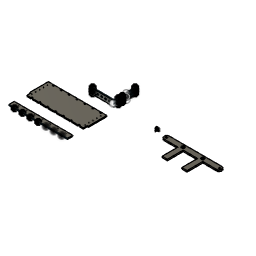
Supporto Netgear v27 (Autodesk Fusion 360 design; units mm, degrees)
Autodesk Fusion 360 part; units mm, degrees
sketch "Schizzo1" plane through (0, 0, 0) normal (0, 0, 1) x (1, 0, 0)
  line L0 (10, 5.25) -> (18, 5.25)
  line L1 (18, 5.25) -> (18, -2.75)
  line L2 (18, -2.75) -> (10, -2.75)
  line L3 (10, -2.75) -> (10, 5.25)
  line L4 (14, 5.25) -> (14, -2.75) construction
  line L5 (10, 1.25) -> (18, 1.25) construction
  circle A0 centre (14, 1.25) radius 2
  line L6 (10, 3.25) -> (18, 3.25) construction
  line L7 (12, 5.25) -> (12, -2.75) construction
  line L8 (12, 5.25) -> (10, 3.25)
  line L9 (16, 5.25) -> (18, 3.25)
  line L10 (16, -2.75) -> (18, -0.75)
  line L11 (12, -2.75) -> (10, -0.75)
  line L12 (21, -0.5) -> (7, -0.5)
  line L13 (7, -0.5) -> (7, 3)
  line L14 (7, 3) -> (21, 3)
  line L15 (21, 3) -> (21, -0.5)
  line L16 (21, -0.5) -> (7, 3) construction
  line L17 (7, -0.5) -> (21, 3) construction
  line L18 (61.544, 0) -> (261.544, 0)
  line L19 (261.544, 0) -> (261.544, -20)
  line L20 (261.544, -20) -> (61.544, -20)
  line L21 (61.544, -20) -> (61.544, 0)
  line L22 (61.544, -10) -> (261.544, -10) construction
  line L23 (124.044, 0) -> (124.044, -20) construction
  line L24 (199.044, 0) -> (199.044, -20) construction
  line L25 (124.044, -10) -> (161.544, -10) construction
  line L26 (161.544, -10) -> (199.044, -10) construction
  circle A1 centre (124.044, -10) radius 3.1
  line L27 (120.944, -10) -> (120.944, -6.9)
  arc A2 (127.144, -6.9) -> (120.944, -6.9) centre (124.044, -6.9) ccw
  line L28 (127.144, -6.9) -> (127.144, -10)
  line L29 (161.544, 0) -> (161.544, -20) construction
  line L30 (124.044, -10) -> (120.944, -10) construction
  line L31 (124.044, -10) -> (127.144, -10) construction
  line L32 (120.944, -10) -> (120.944, -13.1)
  arc A3 (120.944, -13.1) -> (127.144, -13.1) centre (124.044, -13.1) ccw
  line L33 (127.144, -13.1) -> (127.144, -10)
  line L34 (195.944, -13.1) -> (195.944, -10)
  arc A4 (195.944, -13.1) -> (202.144, -13.1) centre (199.044, -13.1) ccw
  line L35 (202.144, -10) -> (202.144, -13.1)
  arc A5 (202.144, -6.9) -> (195.944, -6.9) centre (199.044, -6.9) ccw
  line L36 (202.144, -10) -> (202.144, -6.9)
  line L37 (195.944, -6.9) -> (195.944, -10)
  circle A6 centre (124.044, -10) radius 6.2
  circle A7 centre (199.044, -10) radius 6.2
  circle A8 centre (59.944, -10) radius 3.4
  circle A9 centre (263.144, -10) radius 3.4
  arc A10 (61.544, 0) -> (61.544, -20) centre (61.544, -10) ccw
  arc A11 (261.544, -20) -> (261.544, 0) centre (261.544, -10) ccw
  line L38 (114.044, -20) -> (134.044, -20)
  line L39 (134.044, -20) -> (134.044, -80)
  line L40 (134.044, -80) -> (114.044, -80)
  line L41 (114.044, -80) -> (114.044, -20)
  line L42 (189.044, -20) -> (189.044, -80)
  line L43 (209.044, -80) -> (209.044, -20)
  line L44 (189.044, -80) -> (209.044, -80)
  line L45 (209.044, -20) -> (189.044, -20)
  line L46 (63.994, -5.95) -> (55.894, -5.95)
  line L47 (55.894, -5.95) -> (55.894, -14.05)
  line L48 (55.894, -14.05) -> (63.994, -14.05)
  line L49 (63.994, -14.05) -> (63.994, -5.95)
  line L50 (63.994, -5.95) -> (55.894, -14.05) construction
  line L51 (55.894, -5.95) -> (63.994, -14.05) construction
  line L52 (267.194, -5.95) -> (267.194, -14.05)
  line L53 (267.194, -14.05) -> (259.094, -14.05)
  line L54 (259.094, -14.05) -> (259.094, -5.95)
  line L55 (259.094, -5.95) -> (267.194, -5.95)
  line L56 (-150, 0) -> (-146, 0)
  line L57 (-146, 0) -> (-146, 86)
  line L58 (-146, 86) -> (-150, 86)
  line L59 (-150, 86) -> (-150, 0)
  line L60 (-146, 0) -> (-236, 0)
  line L61 (-236, 0) -> (-236, -4)
  line L62 (-236, -4) -> (-146, -4)
  line L63 (-146, -4) -> (-146, 0)
  line L64 (-150, 15) -> (-165, 0)
  line L65 (-350.1087, -50) -> (-330.1087, -50) construction
  line L66 (-330.1087, -50) -> (-330.1087, -136) construction
  line L67 (-330.1087, -136) -> (-350.1087, -136) construction
  line L68 (-350.1087, -136) -> (-350.1087, -50) construction
  line L69 (-340.1087, -50) -> (-340.1087, -136) construction
  line L70 (-350.1087, -93) -> (-330.1087, -93) construction
  line L71 (-350.1087, -50) -> (-126.9087, -50)
  line L72 (-126.9087, -50) -> (-126.9087, -136)
  line L73 (-126.9087, -136) -> (-350.1087, -136)
  line L74 (-350.1087, -136) -> (-350.1087, -50)
  line L75 (-146.9087, -50) -> (-126.9087, -50) construction
  line L76 (-126.9087, -50) -> (-126.9087, -136) construction
  line L77 (-126.9087, -136) -> (-146.9087, -136) construction
  line L78 (-146.9087, -136) -> (-146.9087, -50) construction
  line L79 (-136.9087, -50) -> (-136.9087, -136) construction
  line L80 (-146.9087, -93) -> (-126.9087, -93) construction
  circle A12 centre (-340.1087, -93) radius 1.4
  line L81 (-330.1087, -78) -> (-350.1087, -78) construction
  line L82 (-330.1087, -63) -> (-350.1087, -63) construction
  circle A13 centre (-340.1087, -78) radius 1.4
  circle A14 centre (-340.1087, -63) radius 1.4
  circle A15 centre (-340.1087, -123) radius 1.4
  circle A16 centre (-340.1087, -108) radius 1.4
  line L83 (-238.5087, -50) -> (-238.5087, -136) construction
  line L84 (-330.1087, -93) -> (-146.9087, -93) construction
  circle A17 centre (-136.9087, -63) radius 1.4
  circle A18 centre (-136.9087, -78) radius 1.4
  circle A19 centre (-136.9087, -93) radius 1.4
  circle A20 centre (-136.9087, -108) radius 1.4
  circle A21 centre (-136.9087, -123) radius 1.4
  line L85 (-350.1087, -134) -> (-126.9087, -134) construction
  line L86 (-268.5087, -136) -> (-268.5087, -50) construction
  line L87 (-298.5087, -136) -> (-298.5087, -50) construction
  line L88 (-328.5087, -50) -> (-328.5087, -136) construction
  circle A22 centre (-328.5087, -134) radius 1.4
  circle A23 centre (-298.5087, -134) radius 1.4
  circle A24 centre (-268.5087, -134) radius 1.4
  circle A25 centre (-238.5087, -134) radius 1.4
  circle A26 centre (-328.5087, -134) radius 3
  circle A27 centre (-298.5087, -134) radius 3
  circle A28 centre (-268.5087, -134) radius 3
  circle A29 centre (-238.5087, -134) radius 3
  circle A30 centre (-148.5087, -134) radius 3
  circle A31 centre (-148.5087, -134) radius 1.4
  circle A32 centre (-178.5087, -134) radius 1.4
  circle A33 centre (-178.5087, -134) radius 3
  circle A34 centre (-208.5087, -134) radius 3
  circle A35 centre (-208.5087, -134) radius 1.4
  circle A36 centre (-328.5087, -52) radius 3
  circle A37 centre (-328.5087, -52) radius 1.4
  circle A38 centre (-298.5087, -52) radius 3
  circle A39 centre (-298.5087, -52) radius 1.4
  circle A40 centre (-268.5087, -52) radius 3
  circle A41 centre (-268.5087, -52) radius 1.4
  circle A42 centre (-238.5087, -52) radius 3
  circle A43 centre (-238.5087, -52) radius 1.4
  circle A44 centre (-208.5087, -52) radius 3
  circle A45 centre (-208.5087, -52) radius 1.4
  circle A46 centre (-178.5087, -52) radius 1.4
  circle A47 centre (-178.5087, -52) radius 3
  circle A48 centre (-148.5087, -52) radius 1.4
  circle A49 centre (-148.5087, -52) radius 3
  line L89 (-350.1087, -121) -> (-126.9087, -121) construction
  line L90 (-350.1087, -121) -> (-346.1087, -121)
  line L91 (-346.1087, -121) -> (-346.1087, -136)
  line L92 (-346.1087, -136) -> (-350.1087, -136)
  line L93 (-350.1087, -136) -> (-350.1087, -121)
  line L94 (-130.9087, -121) -> (-130.9087, -136)
  line L95 (-126.9087, -121) -> (-130.9087, -121)
  line L96 (-350.1087, -180) -> (-126.9087, -180)
  line L97 (-126.9087, -180) -> (-126.9087, -200)
  line L98 (-126.9087, -200) -> (-350.1087, -200)
  line L99 (-350.1087, -200) -> (-350.1087, -180)
  line L100 (-126.9087, -136) -> (-126.9087, -180) construction
  line L101 (-350.1087, -136) -> (-350.1087, -180) construction
  line L102 (15.75, -5.75) -> (12.25, -5.75)
  line L103 (12.25, -5.75) -> (12.25, 8.25)
  line L104 (12.25, 8.25) -> (15.75, 8.25)
  line L105 (15.75, 8.25) -> (15.75, -5.75)
  line L106 (15.75, -5.75) -> (12.25, 8.25) construction
  line L107 (12.25, -5.75) -> (15.75, 8.25) construction
  arc A50 (15.75, 8.25) -> (12.25, 8.25) centre (14, 8.25) ccw
  arc A51 (12.25, -5.75) -> (15.75, -5.75) centre (14, -5.75) ccw
  arc A52 (21, -0.5) -> (21, 3) centre (21, 1.25) ccw
  arc A53 (7, 3) -> (7, -0.5) centre (7, 1.25) ccw
  line L108 (124.044, -20) -> (124.044, -80) construction
  point P0 (14, 1.25)
  point P1 (59.944, -10)
  point P2 (14, 1.25)
  point P3 (124.044, -3.8)
  point P4 (124.044, -16.2)
  dimension "d1" = 8
  dimension "d2" = 8
  dimension "d3" = 4
  dimension "d8" = 2
  dimension "d9" = 2
  dimension "d10" = 14
  dimension "d11" = 3.5
  dimension "d12" = 200
  dimension "d13" = 20
  dimension "d14" = 75
  dimension "d15" = 6.2
  dimension "d28" = 6.8
  dimension "d29" = 101.6
  dimension "d30" = 203.2
  dimension "d31" = 20
  dimension "d32" = 60
  dimension "d63" = 8.1
  dimension "d64" = 8.1
  dimension "d67" = 4
  dimension "d69" = 90
  dimension "d70" = 4
  dimension "d117" = 20
  dimension "d118" = 86
  dimension "d119" = 20
  dimension "d121" = 86
  dimension "d122" = 203.2
  dimension "d125" = 90
  dimension "d126" = 2.8
  dimension "d127" = 15
  dimension "d128" = 15
  dimension "d129" = 2.8
  dimension "d130" = 2.8
  dimension "d131" = 2
  dimension "d132" = 30
  dimension "d133" = 30
  dimension "d134" = 30
  dimension "d135" = 2.8
  dimension "d136" = 2.8
  dimension "d137" = 2.8
  dimension "d138" = 2.8
  dimension "d139" = 6
  dimension "d140" = 6
  dimension "d141" = 6
  dimension "d142" = 6
  dimension "d148" = 15
  dimension "d149" = 15
  dimension "d150" = 15
  dimension "d151" = 4
  dimension "d162" = 20
  dimension "d172" = 3.5
  dimension "d173" = 14
  dimension "d180" = 12.4
  constraint horizontal L0
  constraint vertical L1
  constraint horizontal L2
  constraint vertical L3
  constraint midpoint L0 L4.start
  constraint midpoint L2 L4.end
  constraint midpoint L3 L5.start
  constraint midpoint L1 L5.end
  constraint midpoint L4 P2
  constraint coincident L3 L6.start
  constraint coincident L1 L6.end
  constraint perpendicular L1 L6
  constraint coincident L0 L7.start
  constraint coincident L2 L7.end
  constraint perpendicular L2 L7
  constraint symmetric L4 L6.start L6.end
  constraint symmetric L4 L7.start L9.start
  constraint symmetric L5 L6.start L11.end
  constraint symmetric L5 L7.start L7.end
  constraint symmetric L5 L9.start L10.start
  constraint symmetric L5 L6.end L10.end
  constraint horizontal L12
  constraint perpendicular L12 L13
  constraint parallel L12 L14
  constraint parallel L13 L15
  constraint coincident L16 P2
  constraint coincident L17 P2
  constraint coincident P2 P0
  constraint horizontal L18
  constraint vertical L19
  constraint horizontal L20
  constraint vertical L21
  constraint midpoint L21 L22.start
  constraint midpoint L19 L22.end
  constraint coincident L18 L23.start
  constraint coincident L20 L23.end
  constraint perpendicular L20 L23
  constraint coincident L18 L24.start
  constraint coincident L20 L24.end
  constraint perpendicular L20 L24
  constraint coincident L23 L25.start
  constraint coincident L24 L26.end
  constraint perpendicular L24 L26
  constraint equal L25 L26
  constraint midpoint L23 L25.start
  constraint parallel L23 L27
  constraint tangent L27 A2
  constraint tangent A2 L28
  constraint parallel L23 L28
  constraint coincident L22 L27.start
  constraint coincident A1 L27.start
  constraint tangent A1 L28
  constraint coincident A1 A2.centre
  constraint collinear L22 L25
  constraint midpoint L18 L29.start
  constraint perpendicular L22 L29
  constraint coincident L25.end L29
  constraint coincident L25.start A1.centre
  constraint coincident A1 L28.end
  constraint coincident L22 L28.end
  constraint coincident L28.end L31.end
  constraint symmetric L22 L27.start L30.end
  constraint symmetric L22 L27.end L32.end
  constraint symmetric L22 A2.start A3.end
  constraint symmetric L22 A2 A3
  constraint symmetric L22 L28.end L31.end
  constraint symmetric L27.start L29 L35.start
  constraint symmetric L27.end L29 A5.start
  constraint symmetric A2.start L29 A5.end
  constraint symmetric A2 L29 A5
  constraint symmetric L28.end L29 L34.end
  constraint symmetric L29 L27.start L35.start
  constraint symmetric L29 L32.end A4.end
  constraint symmetric L29 A3.end L34.start
  constraint symmetric L29 A3 A4
  constraint symmetric L29 L28.end L34.end
  constraint tangent A2 A6
  constraint symmetric L29 A6 A7
  constraint coincident L22 P1
  constraint symmetric L29 A8 A9
  constraint tangent L18 A10
  constraint symmetric L18.start L29 L18.end
  constraint symmetric L20.end L29 L19.end
  constraint symmetric L29 A10 A11
  constraint coincident L20 L29.end
  constraint horizontal L38
  constraint vertical L39
  constraint horizontal L40
  constraint vertical L41
  constraint collinear L20 L38
  constraint symmetric L29 L38.start L43.end
  constraint symmetric L29 L38.end L42.start
  constraint symmetric L29 L39.end L42.end
  constraint symmetric L29 L40.end L43.start
  constraint horizontal L46
  constraint perpendicular L46 L47
  constraint parallel L46 L48
  constraint parallel L47 L49
  constraint coincident L50 P1
  constraint coincident L51 P1
  constraint coincident P1 A8.centre
  constraint symmetric L29 L46.start L54.end
  constraint symmetric L29 L46.end L52.start
  constraint symmetric L29 L47.end L52.end
  constraint symmetric L29 L48.end L53.end
  constraint horizontal L56
  constraint vertical L57
  constraint horizontal L58
  constraint vertical L59
  constraint horizontal L60
  constraint vertical L61
  constraint horizontal L62
  constraint vertical L63
  constraint coincident L59 L64.start
  constraint coincident L60 L64.end
  constraint horizontal L65
  constraint vertical L66
  constraint horizontal L67
  constraint vertical L68
  constraint midpoint L65 L69.start
  constraint midpoint L67 L69.end
  constraint midpoint L68 L70.start
  constraint midpoint L66 L70.end
  constraint horizontal L71
  constraint vertical L72
  constraint horizontal L73
  constraint vertical L74
  constraint collinear L67 L73
  constraint horizontal L75
  constraint vertical L76
  constraint horizontal L77
  constraint vertical L78
  constraint midpoint L75 L79.start
  constraint midpoint L77 L79.end
  constraint midpoint L78 L80.start
  constraint midpoint L76 L80.end
  constraint collinear L72 L76
  constraint midpoint L70 A12.centre
  constraint coincident L66 L81.start
  constraint coincident L74 L81.end
  constraint perpendicular L74 L81
  constraint coincident L66 L82.start
  constraint coincident L68 L82.end
  constraint perpendicular L68 L82
  constraint midpoint L81 A13.centre
  constraint midpoint L82 A14.centre
  constraint symmetric L70 A13 A16
  constraint symmetric L70 A14 A15
  constraint midpoint L71 L83.start
  constraint midpoint L73 L83.end
  constraint perpendicular L78 L84
  constraint symmetric A12 L83 A19
  constraint symmetric A13 L83 A18
  constraint symmetric A14 L83 A17
  constraint symmetric A15 L83 A21
  constraint symmetric A16 L83 A20
  constraint coincident L74 L85.start
  constraint coincident L76 L85.end
  constraint perpendicular L76 L85
  constraint coincident L73 L86.start
  constraint coincident L71 L86.end
  constraint perpendicular L71 L86
  constraint coincident L73 L87.start
  constraint coincident L71 L87.end
  constraint perpendicular L71 L87
  constraint coincident L71 L88.start
  constraint coincident L73 L88.end
  constraint perpendicular L73 L88
  constraint coincident L88 A22.centre
  constraint coincident L85 A22.centre
  constraint coincident L87 A23.centre
  constraint coincident L85 A23.centre
  constraint coincident L85 A24.centre
  constraint coincident L86 A24.centre
  constraint midpoint L85 A25.centre
  constraint concentric A22 A26
  constraint concentric A23 A27
  constraint concentric A24 A28
  constraint concentric A25 A29
  constraint symmetric L83 A22 A31
  constraint symmetric L83 A23 A32
  constraint symmetric L83 A24 A35
  constraint symmetric L83 A26 A30
  constraint symmetric L83 A27 A33
  constraint symmetric L83 A28 A34
  constraint symmetric L84 A22 A37
  constraint symmetric L84 A23 A39
  constraint symmetric L84 A24 A41
  constraint symmetric L84 A25 A43
  constraint symmetric L84 A26 A36
  constraint symmetric L84 A27 A38
  constraint symmetric L84 A28 A40
  constraint symmetric L84 A29 A42
  constraint symmetric L84 A30 A49
  constraint symmetric L84 A31 A48
  constraint symmetric L84 A32 A46
  constraint symmetric L84 A33 A47
  constraint symmetric L84 A34 A44
  constraint symmetric L84 A35 A45
  constraint coincident L74 L89.start
  constraint coincident L76 L89.end
  constraint perpendicular L76 L89
  constraint horizontal L90
  constraint vertical L91
  constraint horizontal L92
  constraint vertical L93
  constraint symmetric L83 L89.start L89.end
  constraint symmetric L83 L90.end L94.start
  constraint symmetric L83 L91.end L94.end
  constraint horizontal L96
  constraint vertical L97
  constraint horizontal L98
  constraint vertical L99
  constraint perpendicular L77 L100
  constraint coincident L96.end L97.start
  constraint perpendicular L92 L101
  constraint coincident L96.start L99.end
  constraint horizontal L102
  constraint perpendicular L102 L103
  constraint parallel L102 L104
  constraint parallel L103 L105
  constraint coincident L106 P2
  constraint coincident L107 P2
  constraint tangent L105 A50
  constraint tangent L105 A51
  constraint tangent L14 A52
  constraint tangent L12 A53
  constraint midpoint L38 L23.end
  constraint midpoint L40 L108.end
  constraint collinear L23 L108
  constraint midpoint A2 P3
  constraint midpoint A3 P4
  measures "d1" distance of L0.start L0.end
  measures "d2" distance of L0.start L2.end
  measures "d3" diameter of A0
  measures "d8" distance of L0 L6
  measures "d9" distance of L3 L7
  measures "d10" distance of L13.end L14.end
  measures "d11" distance of L12.end L13.end
  measures "d12" distance of L18.start L18.end
  measures "d13" distance of L18.start L20.end
  measures "d14" distance of L23 L24
  measures "d15" diameter of A1
  measures "d28" diameter of A8
  measures "d29" distance of L29 P1
  measures "d30" distance of P1 A9.centre
  measures "d31" distance of L38.start L38.end
  measures "d32" distance of L38.start L40.end
  measures "d63" distance of L47.end L48.end
  measures "d64" distance of L46.end L47.end
  measures "d67" distance of L56.start L56.end
  measures "d69" distance of L56.end L60.end
  measures "d70" distance of L56.end L62.end
  measures "d117" distance of L65.start L65.end
  measures "d118" distance of L65.start L67.end
  measures "d119" distance of L75.start L71.end
  measures "d121" distance of L71.end L72.end
  measures "d122" distance of L69 L79
  measures "d125" distance of L57.end L62.end
  measures "d126" diameter of A12
  measures "d127" distance of L81 L82
  measures "d128" distance of L70 L81
  measures "d129" diameter of A13
  measures "d130" diameter of A14
  measures "d131" distance of L73 L85
  measures "d132" distance of L83 L86
  measures "d133" distance of L86 L87
  measures "d134" distance of L87 L88
  measures "d135" diameter of A22
  measures "d136" diameter of A23
  measures "d137" diameter of A24
  measures "d138" diameter of A25
  measures "d139" diameter of A26
  measures "d140" diameter of A27
  measures "d141" diameter of A28
  measures "d142" diameter of A29
  measures "d148" distance of L56.start L64.end
  measures "d149" distance of L56.start L64.start
  measures "d150" distance of L67 L89
  measures "d151" distance of L89.start L90.end
  measures "d162" distance of L96.start L98.end
  measures "d172" distance of L103.end L104.end
  measures "d173" distance of L102.end L103.end
  measures "d180" distance of P3 P4
extrude "Estrusione1" add sketch "Schizzo1" along normal blind 2.8 contours L0 L3 L8 L14 L103 | L0 L103 L104 L105 | L0 A0 L14 L103 L105 | L3 A0 L12 L14 L103 | L3 L12 L13 L14 | L0 L1 L9 L14 L105 | A0 L14 L103 | L104 A50 | L2 L3 L11 L12 L103 | L13 A53 | A0 L14 L105 | L1 A0 L12 L14 L105 | A0 L12 L103 | L2 A0 L12 L103 L105 | L1 L12 L14 L15 | L2 L102 L103 L105 | L1 L2 L10 L12 L105 | L15 A52 | A0 L12 L105 | L102 A51 makes body 1
extrude "Estrusione2" add sketch "Schizzo1" along normal blind 6 contours A0 L12 L14 L103 L105 | A0 L14 | A0 L103 | A0 L105 | A0 L12 bodies 1
sketch "Schizzo2" plane through (0, 0, 6) normal (0, 0, 1) x (-1, 0, 0)
  line L0 (-17.5, -0.65) -> (-10.5, -0.65)
  line L1 (-10.5, -0.65) -> (-10.5, -1.85)
  line L2 (-10.5, -1.85) -> (-17.5, -1.85)
  line L3 (-17.5, -1.85) -> (-17.5, -0.65)
  line L4 (-17.5, -0.65) -> (-10.5, -1.85) construction
  line L5 (-10.5, -0.65) -> (-17.5, -1.85) construction
  circle A0 centre (-14, -1.25) radius 3 construction
  circle A1 centre (-14, -1.25) radius 2 construction
  line L6 (-11, -1.25) -> (-11, 1.75) construction
  line L7 (-17, -1.25) -> (-17, 1.75) construction
  line L8 (-11, 1.75) -> (-17, 1.75)
  line L9 (-11, -1.25) -> (-17, -1.25) construction
  line L10 (-14, 1.75) -> (-14.0003, -4.25) construction
  line L11 (-11, -4.25) -> (-17, -4.25)
  arc A2 (-17, 1.75) -> (-17, -4.25) centre (-17, -1.25) ccw
  arc A3 (-11, -4.25) -> (-11, 1.75) centre (-11, -1.25) ccw
  point P0 (-14, -1.25)
  dimension "d24" = 7
  dimension "d25" = 1.2
  dimension "d181" = 6
  constraint horizontal L0
  constraint perpendicular L0 L1
  constraint parallel L0 L2
  constraint parallel L1 L3
  constraint coincident L4 P0
  constraint coincident L5 P0
  constraint concentric A0 A1
  constraint coincident P0 A0.centre
  constraint coincident A0 L6.start
  constraint vertical L6
  constraint coincident A0 L7.start
  constraint vertical L7
  constraint perpendicular L6 L8
  constraint tangent A0 L8
  constraint midpoint L8 L10.start
  constraint coincident A0 L10.end
  constraint symmetric L6.end L9 L11.start
  constraint symmetric L7.end L9 L11.end
  constraint coincident P0 L9
  constraint horizontal L9
  constraint coincident L7.start L9.end
  constraint coincident L6.start L9.start
  measures "d24" distance of L1.end L2.end
  measures "d25" distance of L0.end L1.end
  measures "d181" diameter of A0
extrude "Estrusione4" add sketch "Schizzo2" along normal blind 2.5 bodies 1
extrude "Estrusione6" add sketch "Schizzo2" along normal blind 1 contours L0 L1 L2 L3 bodies 1
extrude "Estrusione3" add sketch "Schizzo1" along normal blind 5 separate body contours L18 L19 L20 L21 L38 L45 L46 L48 L49 L53 L54 L55 | L21 A10 L46 L47 L48 | L19 A11 L52 L53 L55 | L21 A8 L46 L48 L49 | L21 A8 L46 L47 L48 | L19 A9 L52 L53 L55 | L19 A9 L53 L54 L55 | L20 L38 L39 L40 L41 | L20 L42 L43 L44 L45 makes body 2
extrude "Estrusione5" add sketch "Schizzo1" along normal blind 2.2 contours A2 L28 A3 L33 A6 | L27 A2 L32 A3 A6 | L34 A4 A5 L37 A7 | A4 L35 A5 L36 A7 bodies 2
extrude "Estrusione13" cut sketch "Schizzo1" along normal blind 2 contours L21 A8 L46 L48 L49 | L21 A8 L46 L47 L48 | L19 A9 L52 L53 L55 | L19 A9 L53 L54 L55 bodies 2
extrude "Estrusione14" add sketch "Schizzo1" along normal blind 20 separate body contours L56 L57 L58 L59 L60 | L56 L60 L61 L62 L63 makes body 3
extrude "Estrusione15" add sketch "Schizzo1" along normal blind 4 contours L59 L60 L64 bodies 3
sketch "Schizzo7" plane through (-146, 0, 0) normal (1, 0, 0) x (0, 1, 0)
  line L0 (-4, 0) -> (86, 0)
  line L1 (86, 0) -> (86, 20)
  line L2 (86, 20) -> (-4, 20)
  line L3 (-4, 20) -> (-4, 0)
  line L4 (-4, 10) -> (86, 10) construction
  line L5 (43, 20) -> (43, 0) construction
  line L6 (28, 20) -> (28, 0) construction
  line L7 (13, 20) -> (13, 0) construction
  circle A0 centre (13, 10) radius 1.5
  circle A1 centre (28, 10) radius 1.5
  circle A2 centre (43, 10) radius 1.5
  circle A3 centre (13, 10) radius 3
  circle A4 centre (28, 10) radius 3
  circle A5 centre (43, 10) radius 3
  circle A6 centre (58, 10) radius 3
  circle A7 centre (58, 10) radius 1.5
  circle A8 centre (73, 10) radius 3
  circle A9 centre (73, 10) radius 1.5
  line L8 (83.0644, 0.0434) -> (79.0545, -0.0362) construction
  line L9 (79.0545, -0.0362) -> (78.9356, 5.9566) construction
  line L10 (78.9356, 5.9566) -> (82.9455, 6.0362) construction
  line L11 (82.9455, 6.0362) -> (83.0644, 0.0434) construction
  dimension "d91" = 15
  dimension "d92" = 15
  dimension "d93" = 3
  dimension "d94" = 3
  dimension "d95" = 3
  dimension "d96" = 6
  dimension "d97" = 6
  dimension "d98" = 6
  dimension "d124" = 90
  dimension "d154" = 43
  dimension "d155" = 5
  text T0 "1" font "Arial" height 5 align left top in box 4.0107 x 5.9939 at (83.0644, 0.0434) x (-0.999803, -0.019851) y (-0.019851, 0.999803) spacing 1 kerned
  constraint midpoint L3 L4.start
  constraint midpoint L1 L4.end
  constraint coincident L2 L6.start
  constraint coincident L0 L6.end
  constraint perpendicular L0 L6
  constraint coincident L2 L7.start
  constraint coincident L0 L7.end
  constraint perpendicular L0 L7
  constraint midpoint L7 A0.centre
  constraint midpoint L6 A1.centre
  constraint midpoint L5 A2.centre
  constraint concentric A0 A3
  constraint concentric A1 A4
  constraint concentric A2 A5
  constraint symmetric L5 A0 A9
  constraint symmetric L5 A1 A7
  constraint symmetric L5 A3 A8
  constraint symmetric L5 A4 A6
  measures "d91" distance of L6 L7
  measures "d92" distance of L5 L6
  measures "d93" diameter of A0
  measures "d94" diameter of A1
  measures "d95" diameter of A2
  measures "d96" diameter of A3
  measures "d97" diameter of A4
  measures "d98" diameter of A5
  measures "d124" distance of L1 L3
  measures "d154" distance of L4.end L5
sketch "Schizzo8" plane through (0, 0, 0) normal (0, 1, 0) x (-1, 0, 0)
  line L0 (165, 4) -> (165, 0)
  line L1 (165, 0) -> (236, 0)
  line L2 (236, 0) -> (236, 20)
  line L3 (236, 20) -> (150, 20)
  line L4 (150, 20) -> (150, 4)
  line L5 (150, 4) -> (165, 4)
  line L6 (236, 10) -> (146, 10) construction
  line L7 (231, 0) -> (231, 20) construction
  line L8 (226.95, 14.05) -> (235.05, 14.05)
  line L9 (235.05, 14.05) -> (235.05, 5.95)
  line L10 (235.05, 5.95) -> (226.95, 5.95)
  line L11 (226.95, 5.95) -> (226.95, 14.05)
  line L12 (226.95, 14.05) -> (235.05, 5.95) construction
  line L13 (235.05, 14.05) -> (226.95, 5.95) construction
  circle A0 centre (231, 10) radius 3.4
  point P0 (231, 10)
  dimension "d75" = 8.1
  dimension "d76" = 8.1
  dimension "d77" = 6.8
  dimension "d82" = 5
  constraint midpoint L2 L6.start
  constraint perpendicular L4 L6
  constraint coincident L1 L7.start
  constraint coincident L3 L7.end
  constraint perpendicular L3 L7
  constraint horizontal L8
  constraint perpendicular L8 L9
  constraint parallel L8 L10
  constraint parallel L9 L11
  constraint coincident L12 P0
  constraint coincident L13 P0
  constraint midpoint L7 P0
  constraint coincident P0 A0.centre
  measures "d75" distance of L9.end L10.end
  measures "d76" distance of L8.end L9.end
  measures "d77" diameter of A0
  measures "d82" distance of L2 L7
extrude "Estrusione16" cut sketch "Schizzo8" against normal blind 4 contours A0 bodies 3
extrude "Estrusione17" cut sketch "Schizzo8" against normal blind 2 contours L8 L9 L10 L11 bodies 3
sketch "Schizzo9" plane through (-150, 0, 0) normal (-1, 0, 0) x (0, -1, 0)
  line L0 (-15, 4) -> (0, 4)
  line L1 (0, 4) -> (0, 20)
  line L2 (0, 20) -> (-86, 20)
  line L3 (-86, 20) -> (-86, 0)
  line L4 (-86, 0) -> (-15, 0)
  line L5 (-15, 0) -> (-15, 4)
  line L6 (-86, 10) -> (4, 10) construction
  line L7 (-81, 0) -> (-81, 20) construction
  line L8 (-85.05, 5.95) -> (-76.95, 5.95)
  line L9 (-76.95, 5.95) -> (-76.95, 14.05)
  line L10 (-76.95, 14.05) -> (-85.05, 14.05)
  line L11 (-85.05, 14.05) -> (-85.05, 5.95)
  line L12 (-85.05, 5.95) -> (-76.95, 14.05) construction
  line L13 (-76.95, 5.95) -> (-85.05, 14.05) construction
  circle A0 centre (-81, 10) radius 3.4
  point P0 (-81, 10)
  dimension "d83" = 8.1
  dimension "d84" = 8.1
  dimension "d85" = 6.8
  dimension "d90" = 5
  constraint midpoint L3 L6.start
  constraint perpendicular L1 L6
  constraint coincident L4 L7.start
  constraint coincident L2 L7.end
  constraint perpendicular L2 L7
  constraint horizontal L8
  constraint perpendicular L8 L9
  constraint parallel L8 L10
  constraint parallel L9 L11
  constraint coincident L12 P0
  constraint coincident L13 P0
  constraint midpoint L7 P0
  constraint coincident P0 A0.centre
  measures "d83" distance of L9.end L10.end
  measures "d84" distance of L8.end L9.end
  measures "d85" diameter of A0
  measures "d90" distance of L3 L7
extrude "Estrusione20" cut sketch "Schizzo7" against normal blind 4 contours A0 | A1 | A2 | A7 | A9 bodies 3
extrude "Estrusione21" cut sketch "Schizzo7" against normal blind 3.2 contours A3 | A4 | A5 | A6 | A8 bodies 3
extrude "Estrusione18" cut sketch "Schizzo9" against normal blind 4 contours A0 bodies 3
extrude "Estrusione19" cut sketch "Schizzo9" against normal blind 2 contours L8 L9 L10 L11 bodies 3
sketch "Schizzo10" plane through (0, -4, 0) normal (0, -1, 0) x (1, 0, 0)
  circle A0 centre (-231, 10) radius 3.4
  line L0 (-236, 0) -> (-146, 0)
  line L1 (-146, 0) -> (-146, 20)
  line L2 (-146, 20) -> (-236, 20)
  line L3 (-236, 20) -> (-236, 0)
  line L4 (-236, 10) -> (-146, 10) construction
  line L5 (-193, 20) -> (-193, 0) construction
  line L6 (-178, 20) -> (-178, 0) construction
  line L7 (-163, 20) -> (-163, 0) construction
  circle A1 centre (-193, 10) radius 1.5
  circle A2 centre (-178, 10) radius 1.5
  circle A3 centre (-163, 10) radius 1.5
  circle A4 centre (-193, 10) radius 3
  circle A5 centre (-178, 10) radius 3
  circle A6 centre (-163, 10) radius 3
  circle A7 centre (-208, 10) radius 3
  circle A8 centre (-208, 10) radius 1.5
  circle A9 centre (-223, 10) radius 3
  circle A10 centre (-223, 10) radius 1.5
  line L8 (-236, 10) -> (-150, 10)
  line L9 (-217.5306, 1.0257) -> (-212.5287, 0.9763) construction
  line L10 (-212.5287, 0.9763) -> (-212.4694, 6.9743) construction
  line L11 (-212.4694, 6.9743) -> (-217.4713, 7.0237) construction
  line L12 (-217.4713, 7.0237) -> (-217.5306, 1.0257) construction
  point P0 (-150, 10)
  point P1 (-146, 10)
  dimension "d103" = 15
  dimension "d104" = 15
  dimension "d105" = 3
  dimension "d106" = 3
  dimension "d107" = 3
  dimension "d108" = 6
  dimension "d109" = 6
  dimension "d110" = 6
  dimension "d115" = 86
  dimension "d116" = 20
  dimension "d123" = 90
  dimension "d156" = 5
  dimension "d157" = 43
  text T0 "2" font "Arial" height 5 align left top in box 5.0021 x 5.9984 at (-217.5306, 1.0257) x (0.999951, -0.009881) y (0.009881, 0.999951) spacing 1 kerned
  constraint midpoint L3 L4.start
  constraint midpoint L1 P1
  constraint coincident L2 L6.start
  constraint coincident L0 L6.end
  constraint perpendicular L0 L6
  constraint coincident L2 L7.start
  constraint coincident L0 L7.end
  constraint perpendicular L0 L7
  constraint midpoint L5 A1.centre
  constraint midpoint L6 A2.centre
  constraint midpoint L7 A3.centre
  constraint concentric A1 A4
  constraint concentric A2 A5
  constraint concentric A3 A6
  constraint symmetric L5 A2 A8
  constraint symmetric L5 A3 A10
  constraint symmetric L5 A5 A7
  constraint symmetric L5 A6 A9
  constraint coincident L4 P0
  constraint perpendicular L7 L8
  measures "d103" distance of L5 L6
  measures "d104" distance of L6 L7
  measures "d105" diameter of A1
  measures "d106" diameter of A2
  measures "d107" diameter of A3
  measures "d108" diameter of A4
  measures "d109" diameter of A5
  measures "d110" diameter of A6
  measures "d115" horizontal distance of L0.start P0
  measures "d116" distance of L0 L2
  measures "d123" distance of L3 P1
  measures "d157" distance of L3 L5
extrude "Estrusione22" cut sketch "Schizzo10" against normal blind 4 contours A1 L8 | A1 L8 | A2 L8 | A2 L8 | A3 L8 | A3 L8 | A8 L8 | A8 L8 | A10 L8 | A10 L8 bodies 3
extrude "Estrusione23" cut sketch "Schizzo10" against normal blind 2 contours A1 A4 L8 | A1 A4 L8 | A2 A5 L8 | A2 A5 L8 | A3 A6 L8 | A3 A6 L8 | A7 A8 L8 | A7 A8 L8 | A9 A10 L8 | A9 A10 L8 bodies 3
extrude "Estrusione24" add sketch "Schizzo1" along normal blind 4 separate body contours L71 L72 L73 L74 A26 A27 A28 A29 A30 A33 A34 A36 A38 A40 A42 A44 A47 A49 L90 L91 L94 L95 | L96 L97 L98 L99 makes body 4 at (-164.9438, -92.9232, 0) makes body 5 at (-275.7087, -193.3333, 0)
extrude "Estrusione25" add sketch "Schizzo1" along normal blind 0.8 from surface at 3.2 contours L71 A36 | L71 A38 | L73 A26 | L71 A40 | L73 A27 | L71 A42 | L73 A28 | L71 A44 | L73 A29 | L71 A47 | L73 A34 | L71 A49 | L73 A33 | L73 A30 picked at (-328.5435, -50.2013) picked at (-298.5435, -50.2013) picked at (-328.5435, -135.7987) picked at (-268.5435, -50.2013) picked at (-298.5435, -135.7987) picked at (-238.5435, -50.2013) picked at (-268.5435, -135.7987) picked at (-208.5435, -50.2013) picked at (-238.5435, -135.7987) picked at (-178.5435, -50.2013) picked at (-208.5435, -135.7987) picked at (-148.5435, -50.2013) picked at (-178.5435, -135.7987) picked at (-148.5435, -135.7987) bodies 4
extrude "Estrusione26" cut sketch "Schizzo10" against normal blind 1 text T0 bodies 3
extrude "Estrusione27" cut sketch "Schizzo7" against normal blind 1 text T0 bodies 3
sketch "Schizzo11" plane through (0, -200, 0) normal (0, -1, 0) x (1, 0, 0)
  line L0 (-350.1087, 0) -> (-126.9087, 0)
  line L1 (-126.9087, 0) -> (-126.9087, 4)
  line L2 (-126.9087, 4) -> (-350.1087, 4)
  line L3 (-350.1087, 4) -> (-350.1087, 0)
  line L4 (-238.5087, 4) -> (-238.5087, 0) construction
  line L5 (-350.1087, 2) -> (-126.9087, 2) construction
  circle A0 centre (-238.5087, 2) radius 1.4
  circle A1 centre (-268.5087, 2) radius 1.4
  circle A2 centre (-328.5087, 2) radius 1.4
  circle A3 centre (-298.5087, 2) radius 1.4
  circle A4 centre (-148.5087, 2) radius 1.4
  circle A5 centre (-178.5087, 2) radius 1.4
  circle A6 centre (-208.5087, 2) radius 1.4
  dimension "d163" = 2.8
  dimension "d164" = 2.8
  dimension "d165" = 2.8
  dimension "d166" = 2.8
  dimension "d167" = 30
  dimension "d168" = 30
  dimension "d169" = 30
  constraint midpoint L2 L4.start
  constraint midpoint L0 L4.end
  constraint midpoint L3 L5.start
  constraint midpoint L1 L5.end
  constraint midpoint L4 A0.centre
  constraint coincident L5 A1.centre
  constraint coincident L5 A2.centre
  constraint coincident L5 A3.centre
  constraint symmetric L4 A1 A6
  constraint symmetric L4 A2 A4
  constraint symmetric L4 A3 A5
  measures "d163" diameter of A0
  measures "d164" diameter of A1
  measures "d165" diameter of A2
  measures "d166" diameter of A3
  measures "d167" distance of A0.centre A1.centre
  measures "d168" distance of A1.centre A3.centre
  measures "d169" distance of A2.centre A3.centre
extrude "Estrusione28" cut sketch "Schizzo11" against normal blind 15 contours A0 | A1 | A2 | A3 | A4 | A5 | A6 bodies 5
equation "d10 = d173"
equation "d11 = d172"
equation "d29 = ( 25.4 * 4 ) * 1 mm"
equation "d63 = d64"
equation "d67 = d70"
equation "d92 = d91"
equation "d125 = d69"
equation "d127 = d128"
equation "d133 = d132"
equation "d134 = d132"
equation "d164 = d163"
equation "d165 = d163"
equation "d166 = d163"
equation "d168 = d167"
equation "d169 = d167"
named bodies: "Hook", "Frame", "Staffa", "Piano", "Parapetto"
